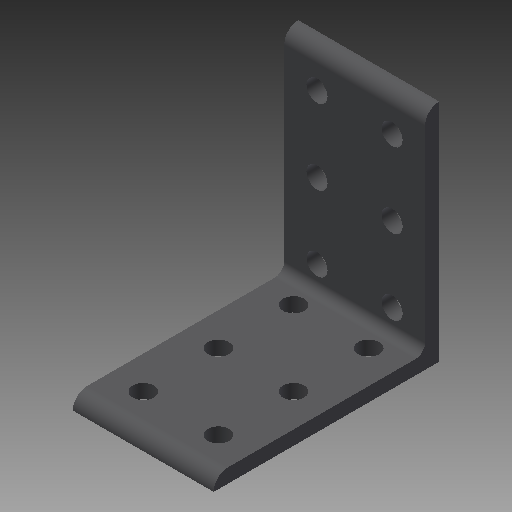
# Autodesk Inventor part: 4014
Saved by Autodesk Inventor 2017 (Build 210142000, 142)
## iProperties
Category: PARTsolutions
Company: 8020
Created: 2017-04-25
Part Number: 4014
Catalog Web Link: www.cadenas.de
Description: 4014, 4414-Joining Plates - 12 Hole Inside Corner Bracket
Vendor: 8020
Document SubType Name: Modeling
Designer: psAdmin
Manufacturer: 8020
Mass: 30.9169 g
Surface Area: 159.752 cm^2
Volume: 30.9169 cm^3
Density: 1 g/cm^3
Material: Generic
Appearance: PSOLRGB-175-175-175
PSOL_IDENT_0: {$CADENAS_DATA\23d-libs\8020\inch\joining_plates\4014.prj},145 {VTYP=3D},{NB=4014},{LINA=4014},{NN=4
PSOL_IDENT_1: 014, 4414},{DATE=22.08.2012},{GEOMDATE=14.12.2011 11:54:00},{VERSION=},{LINEID=10},{LINESUBID=-1},{W
PSOL_IDENT_2: BVAR=}  {NB=4014},{LINA=4014},{KT=DUMMY},{PN=4014},{A=1.875},{B=3.000},{C=3.000},{E=0.281},{W=.176},
PSOL_IDENT_3: {A1=0.4375},{C1=0.500},{C2=1.500},{C3=2.500},{D1=0.188},{R=0.125}
NN: 4014, 4414
NT: Joining Plates - 12 Hole Inside Corner Bracket
NB: 4014
NBSYN: $PN.
LINA: 4014
PN: 4014
A: 1.875
B: 3.000
C: 3.000
W: .176
SUPPLIER: 8020
ARTICLENO: 4014
BOMINFO: 4014
CREATOR: CADENAS GmbH
Title: 4014
Author: Cadenas PARTsolutions
Comments: Joining Plates - 12 Hole Inside Corner Bracket
Autodesk Inventor part; units mm, degrees
ref_plane "YZ Plane" through (0, 0, 0) normal (1, 0, 0) x (0, 1, 0)
ref_plane "XZ Plane" through (0, 0, 0) normal (0, 1, 0) x (-1, 0, 0)
ref_plane "XY Plane" through (0, 0, 0) normal (0, 0, 1) x (1, 0, 0)
sketch "Sketch_1" plane through (0, 0, 0) normal (1, 0, 0) x (0, 1, 0)
  line L0 (0, 76.2) -> (0, 0)
  line L1 (0, 0) -> (76.2, 0)
  arc A0 (76.2, 0) -> (71.4248, 4.7752) centre (71.4248, 0) ccw
  line L2 (71.4248, 4.7752) -> (7.9502, 4.7752)
  arc A1 (4.7752, 7.9502) -> (7.9502, 4.7752) centre (7.9502, 7.9502) ccw
  line L3 (4.7752, 7.9502) -> (4.7752, 71.4248)
  arc A2 (4.7752, 71.4248) -> (0, 76.2) centre (0, 71.4248) ccw
  constraints: 8 end point, 6 point on circle, 3 centre point
extrude "Extrusion1" add sketch "Sketch_1" along normal mid plane 47.625
sketch "Sketch2" plane through (23.8125, 0, 0) normal (0, 0, -1) x (-1, 0, 0)
  point P0 (11.1125, 63.5)
hole "Hole1" at (12.7, 63.5, 0) direction (0, 0, 1) diameter 7.1374 depth 5.2527
sketch "Sketch3" plane through (23.8125, 0, 0) normal (0, 0, -1) x (-1, 0, 0)
  point P0 (36.5125, 38.1)
hole "Hole2" at (-12.7, 38.1, 0) direction (0, 0, 1) diameter 7.1374 depth 5.2527
sketch "Sketch4" plane through (23.8125, 0, 0) normal (0, 0, -1) x (-1, 0, 0)
  point P0 (36.5125, 63.5)
hole "Hole3" at (-12.7, 63.5, 0) direction (0, 0, 1) diameter 7.1374 depth 5.2527
sketch "Sketch5" plane through (-23.8125, 0, 76.2) normal (0, -1, 0) x (1, 0, 0)
  point P0 (36.5125, -38.1)
hole "Hole4" at (12.7, 0, 38.1) direction (0, 1, 0) diameter 7.1374 depth 5.2527
sketch "Sketch6" plane through (-23.8125, 0, 76.2) normal (0, -1, 0) x (1, 0, 0)
  point P0 (36.5125, -12.7)
hole "Hole5" at (12.7, 0, 63.5) direction (0, 1, 0) diameter 7.1374 depth 5.2527
sketch "Sketch7" plane through (-23.8125, 0, 76.2) normal (0, -1, 0) x (1, 0, 0)
  point P0 (11.1125, -38.1)
hole "Hole6" at (-12.7, 0, 38.1) direction (0, 1, 0) diameter 7.1374 depth 5.2527
sketch "Sketch8" plane through (-23.8125, 0, 76.2) normal (0, -1, 0) x (1, 0, 0)
  point P0 (11.1125, -12.7)
hole "Hole7" at (-12.7, 0, 63.5) direction (0, 1, 0) diameter 7.1374 depth 5.2527
sketch "Sketch9" plane through (23.8125, 0, 0) normal (0, 0, -1) x (-1, 0, 0)
  point P0 (11.1125, 38.1)
hole "Hole8" at (12.7, 38.1, 0) direction (0, 0, 1) diameter 7.1374 depth 5.2527
sketch "Sketch10" plane through (23.8125, 0, 0) normal (0, 0, -1) x (-1, 0, 0)
  point P0 (11.1125, 12.7)
hole "Hole9" at (12.7, 12.7, 0) direction (0, 0, 1) diameter 7.1374 depth 5.2527
sketch "Sketch11" plane through (23.8125, 0, 0) normal (0, 0, -1) x (-1, 0, 0)
  point P0 (36.5125, 12.7)
hole "Hole10" at (-12.7, 12.7, 0) direction (0, 0, 1) diameter 7.1374 depth 5.2527
sketch "Sketch12" plane through (-23.8125, 0, 76.2) normal (0, -1, 0) x (1, 0, 0)
  point P0 (36.5125, -63.5)
hole "Hole11" at (12.7, 0, 12.7) direction (0, 1, 0) diameter 7.1374 depth 5.2527
sketch "Sketch13" plane through (-23.8125, 0, 76.2) normal (0, -1, 0) x (1, 0, 0)
  point P0 (11.1125, -63.5)
hole "Hole12" at (-12.7, 0, 12.7) direction (0, 1, 0) diameter 7.1374 depth 5.2527
body "Solid1"
